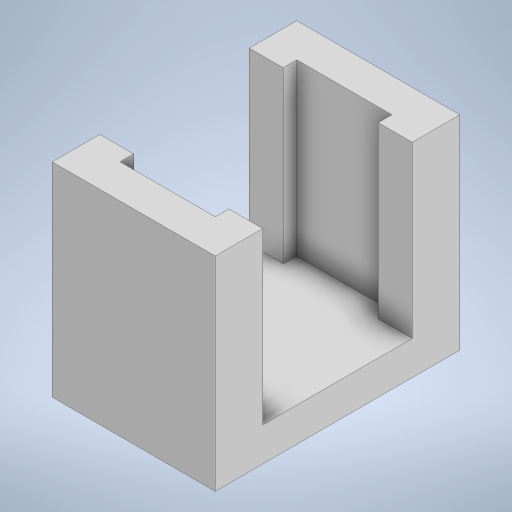
# Autodesk Inventor part: LatchSingleFit
Saved by Autodesk Inventor 2024 (Build 280153000, 153)
## iProperties
Created: 2023-10-31
Part Number: LatchSingleFit
Material: Generic
Document SubType Name: Modeling
Designer: gcter
Density: 1 g/cm^3
Appearance: Default
Author: gcter
Autodesk Inventor part; units mm, degrees
ref_plane "YZ Plane" through (0, 0, 0) normal (1, 0, 0) x (0, 1, 0)
ref_plane "XZ Plane" through (0, 0, 0) normal (0, 1, 0) x (-1, 0, 0)
ref_plane "XY Plane" through (0, 0, 0) normal (0, 0, 1) x (1, 0, 0)
sketch "Sketch5" plane through (0, 0, 0) normal (0, 1, 0) x (-1, 0, 0)
  line L0 (0, 0) -> (-6.604, 0) construction
  line L1 (-6.604, 0) -> (-6.604, -12.7) construction
  line L2 (-6.604, -12.7) -> (0, -12.7) construction
  line L3 (0, -12.7) -> (0, 0) construction
  line L4 (2.794, -15.494) -> (-9.398, -15.494)
  line L5 (-9.398, -15.494) -> (-9.398, 2.794)
  line L6 (-9.398, 2.794) -> (2.794, 2.794)
  line L7 (2.794, 2.794) -> (2.794, -15.494)
  dimension "d22" = 6.604
  dimension "d23" = 12.7
  dimension "d24" = 2.794
  dimension "d25" = 2.794
  dimension "d26" = 2.794
  dimension "d27" = 2.794
  constraints: 16 end point, 4 parallel, 2 horizontal, 2 perpendicular
  measures "d22" distance between parallel lines of L1 L3
  measures "d23" distance between parallel lines of L0 L2
  measures "d24" distance between parallel lines of L5 L1
  measures "d25" distance between parallel lines of L3 L7
  measures "d26" distance between parallel lines of L6 L0
  measures "d27" distance between parallel lines of L2 L4
extrude "Extrusion3" add sketch "Sketch5" along normal blind 2.54
sketch "Sketch6" plane through (0, 2.54, 0) normal (0, 1, 0) x (1, 0, 0)
  line L0 (-2.794, -2.794) -> (9.398, -2.794)
  line L1 (9.398, -2.794) -> (9.398, -0.254)
  line L2 (6.858, -0.254) -> (-0.254, -0.254)
  line L3 (-2.794, -0.254) -> (-2.794, -2.794)
  line L4 (-2.794, 15.494) -> (-2.794, -2.794) projected
  line L5 (9.398, -2.794) -> (9.398, 15.494) projected
  line L6 (-2.794, -2.794) -> (9.398, -2.794) projected
  line L7 (-0.254, 12.954) -> (6.858, 12.954)
  line L8 (9.398, 12.954) -> (9.398, 15.494)
  line L9 (9.398, 15.494) -> (-2.794, 15.494)
  line L10 (-2.794, 15.494) -> (-2.794, 12.954)
  line L11 (9.398, 15.494) -> (-2.794, 15.494) projected
  line L12 (9.398, 12.954) -> (9.398, 11.938)
  line L13 (6.858, 11.938) -> (6.858, 12.954)
  line L14 (6.858, 11.938) -> (9.398, 11.938)
  line L15 (-2.794, 12.954) -> (-2.794, 11.938)
  line L16 (-2.794, 11.938) -> (-0.254, 11.938)
  line L17 (-0.254, 11.938) -> (-0.254, 12.954)
  line L18 (9.398, -0.254) -> (9.398, 0.762)
  line L19 (9.398, 0.762) -> (6.858, 0.762)
  line L20 (6.858, 0.762) -> (6.858, -0.254)
  line L21 (-0.254, -0.254) -> (-0.254, 0.762)
  line L22 (-0.254, 0.762) -> (-2.794, 0.762)
  line L23 (-2.794, 0.762) -> (-2.794, -0.254)
  point P0 (0, 0)
  point P1 (8.128, 11.938)
  point P2 (9.398, 0.254)
  point P3 (9.398, -0.254)
  dimension "d30" = 2.54
  dimension "d31" = 2.54
  dimension "d32" = 2.54
  dimension "d33" = 1.016
  dimension "d35" = 2.54
  dimension "d36" = 1.016
  dimension "d37" = 1.016
  dimension "d38" = 2.54
  dimension "d39" = 2.54
  dimension "d40" = 1.016
  constraints: 40 end point, 9 collinear, 7 parallel, 4 perpendicular, 2 horizontal, 2 midpoint, 1 point on line
  measures "d30" distance between parallel lines of L2 L0
  measures "d31" distance between parallel lines of L7 L9
  measures "d32" distance between parallel lines of L5 L13
  measures "d33" distance from line of L7 point (8.128, 11.938)
  measures "d35" distance between parallel lines of L17 L4
  measures "d36" distance between parallel lines of L7 L16
  measures "d37" distance between parallel lines of L2 L19
  measures "d38" distance from line of point (9.398, 0.254) L20
  measures "d39" distance between parallel lines of L21 L23
  measures "d40" distance between parallel lines of L2 L22
extrude "Extrusion4" add sketch "Sketch6" along normal blind 12.7 contours L3 L4 L22 L21 L2 L20 L19 L5 L1 L0 | L4 L9 L5 L14 L13 L7 L17 L16
body "Solid3"
